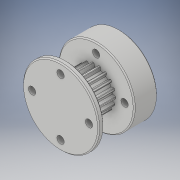
# Autodesk Inventor part: 000.404 - Проставка шкива
Saved by Autodesk Inventor 2019 (Build 230136000, 136)
## iProperties
Created: 2020-03-31
Part Number: 000.404 - Проставка шкива
Material: Типовые
Document SubType Name: Modeling
Designer: Петров Иван
Density: 1 g/cm^3
Appearance: По умолчанию
Author: Петров Иван
Autodesk Inventor part; units mm, degrees
ref_plane "YZ Plane" through (0, 0, 0) normal (1, 0, 0) x (0, 1, 0)
ref_plane "XZ Plane" through (0, 0, 0) normal (0, 1, 0) x (-1, 0, 0)
ref_plane "XY Plane" through (0, 0, 0) normal (0, 0, 1) x (1, 0, 0)
sketch "Эскиз1" plane through (0, 0, 0) normal (0, 0, 1) x (1, 0, 0)
  circle A0 centre (0, -2.75) radius 10.7 projected
  circle A1 centre (0, 5.25) radius 1.025 projected
  circle A2 centre (8, -2.75) radius 1.025 projected
  circle A3 centre (0, -10.75) radius 1.025 projected
  circle A4 centre (-8, -2.75) radius 1.025 projected
  circle A5 centre (0, -2.75) radius 3.05 projected
  point P0 (0, 0)
extrude "Выдавливание1" add sketch "Эскиз1" along normal blind 6.55
sketch "Эскиз2" plane through (0, -2.75, 6.55) normal (0, 0, 1) x (1, 0, 0)
  circle A0 centre (0, 0) radius 7.7
  line L0 (1.9221, 4.23) -> (2.4672, 4.8795)
  arc A1 (2.6243, 4.9099) -> (2.4672, 4.8795) centre (2.5644, 4.7979) ccw
  arc A2 (2.94, 4.7277) -> (2.6243, 4.9099) centre (0, 0) ccw
  arc A3 (2.9922, 4.5764) -> (2.94, 4.7277) centre (2.8729, 4.6198) ccw
  line L1 (2.9922, 4.5764) -> (2.7022, 3.7796)
  line L2 (2.7022, 3.7796) -> (3.2529, 3.3175)
  line L3 (3.2529, 3.3175) -> (3.9873, 3.7415)
  arc A4 (4.1453, 3.7162) -> (3.9873, 3.7415) centre (4.0508, 3.6315) ccw
  arc A5 (4.3796, 3.437) -> (4.1453, 3.7162) centre (0, 0) ccw
  arc A6 (4.377, 3.277) -> (4.3796, 3.437) centre (4.2797, 3.3586) ccw
  line L4 (4.377, 3.277) -> (3.8319, 2.6274)
  line L5 (3.8319, 2.6274) -> (4.1914, 2.0048)
  line L6 (4.1914, 2.0048) -> (5.0265, 2.1521)
  arc A7 (5.1664, 2.0743) -> (5.0265, 2.1521) centre (5.0485, 2.027) ccw
  arc A8 (5.291, 1.7318) -> (5.1664, 2.0743) centre (0, 0) ccw
  arc A9 (5.2338, 1.5823) -> (5.291, 1.7318) centre (5.1703, 1.6923) ccw
  line L7 (5.2338, 1.5823) -> (4.4995, 1.1584)
  line L8 (4.4995, 1.1584) -> (4.6243, 0.4504)
  line L9 (4.6243, 0.4504) -> (5.4594, 0.3032)
  arc A10 (5.5643, 0.1822) -> (5.4594, 0.3032) centre (5.4373, 0.1781) ccw
  arc A11 (5.5643, -0.1822) -> (5.5643, 0.1822) centre (0, 0) ccw
  arc A12 (5.4594, -0.3032) -> (5.5643, -0.1822) centre (5.4373, -0.1781) ccw
  line L10 (5.4594, -0.3032) -> (4.6243, -0.4504)
  line L11 (4.6243, -0.4504) -> (4.4995, -1.1584)
  line L12 (4.4995, -1.1584) -> (5.2338, -1.5823)
  arc A13 (5.291, -1.7318) -> (5.2338, -1.5823) centre (5.1703, -1.6923) ccw
  arc A14 (5.1664, -2.0743) -> (5.291, -1.7318) centre (0, 0) ccw
  arc A15 (5.0265, -2.1521) -> (5.1664, -2.0743) centre (5.0485, -2.027) ccw
  line L13 (5.0265, -2.1521) -> (4.1914, -2.0048)
  line L14 (4.1914, -2.0048) -> (3.8319, -2.6274)
  line L15 (3.8319, -2.6274) -> (4.377, -3.277)
  arc A16 (4.3796, -3.437) -> (4.377, -3.277) centre (4.2797, -3.3586) ccw
  arc A17 (4.1453, -3.7162) -> (4.3796, -3.437) centre (0, 0) ccw
  arc A18 (3.9873, -3.7415) -> (4.1453, -3.7162) centre (4.0508, -3.6315) ccw
  line L16 (3.9873, -3.7415) -> (3.2529, -3.3175)
  line L17 (3.2529, -3.3175) -> (2.7022, -3.7796)
  line L18 (2.7022, -3.7796) -> (2.9922, -4.5764)
  arc A19 (2.94, -4.7277) -> (2.9922, -4.5764) centre (2.8729, -4.6198) ccw
  arc A20 (2.6243, -4.9099) -> (2.94, -4.7277) centre (0, 0) ccw
  arc A21 (2.4672, -4.8795) -> (2.6243, -4.9099) centre (2.5644, -4.7979) ccw
  line L19 (2.4672, -4.8795) -> (1.9221, -4.23)
  line L20 (1.9221, -4.23) -> (1.2466, -4.4758)
  line L21 (1.2466, -4.4758) -> (1.2466, -5.3238)
  arc A22 (1.1457, -5.4481) -> (1.2466, -5.3238) centre (1.1196, -5.3238) ccw
  arc A23 (0.7868, -5.5114) -> (1.1457, -5.4481) centre (0, 0) ccw
  arc A24 (0.6495, -5.4291) -> (0.7868, -5.5114) centre (0.7688, -5.3857) ccw
  line L22 (0.6495, -5.4291) -> (0.3594, -4.6323)
  line L23 (0.3594, -4.6323) -> (-0.3594, -4.6323)
  line L24 (-0.3594, -4.6323) -> (-0.6495, -5.4291)
  arc A25 (-0.7868, -5.5114) -> (-0.6495, -5.4291) centre (-0.7688, -5.3857) ccw
  arc A26 (-1.1457, -5.4481) -> (-0.7868, -5.5114) centre (0, 0) ccw
  arc A27 (-1.2466, -5.3238) -> (-1.1457, -5.4481) centre (-1.1196, -5.3238) ccw
  line L25 (-1.2466, -5.3238) -> (-1.2466, -4.4758)
  line L26 (-1.2466, -4.4758) -> (-1.9221, -4.23)
  line L27 (-1.9221, -4.23) -> (-2.4672, -4.8795)
  arc A28 (-2.6243, -4.9099) -> (-2.4672, -4.8795) centre (-2.5644, -4.7979) ccw
  arc A29 (-2.94, -4.7277) -> (-2.6243, -4.9099) centre (0, 0) ccw
  arc A30 (-2.9922, -4.5764) -> (-2.94, -4.7277) centre (-2.8729, -4.6198) ccw
  line L28 (-2.9922, -4.5764) -> (-2.7022, -3.7796)
  line L29 (-2.7022, -3.7796) -> (-3.2529, -3.3175)
  line L30 (-3.2529, -3.3175) -> (-3.9873, -3.7415)
  arc A31 (-4.1453, -3.7162) -> (-3.9873, -3.7415) centre (-4.0508, -3.6315) ccw
  arc A32 (-4.3796, -3.437) -> (-4.1453, -3.7162) centre (0, 0) ccw
  arc A33 (-4.377, -3.277) -> (-4.3796, -3.437) centre (-4.2797, -3.3586) ccw
  line L31 (-4.377, -3.277) -> (-3.8319, -2.6274)
  line L32 (-3.8319, -2.6274) -> (-4.1914, -2.0048)
  line L33 (-4.1914, -2.0048) -> (-5.0265, -2.1521)
  arc A34 (-5.1664, -2.0743) -> (-5.0265, -2.1521) centre (-5.0485, -2.027) ccw
  arc A35 (-5.291, -1.7318) -> (-5.1664, -2.0743) centre (0, 0) ccw
  arc A36 (-5.2338, -1.5823) -> (-5.291, -1.7318) centre (-5.1703, -1.6923) ccw
  line L34 (-5.2338, -1.5823) -> (-4.4995, -1.1584)
  line L35 (-4.4995, -1.1584) -> (-4.6243, -0.4504)
  line L36 (-4.6243, -0.4504) -> (-5.4594, -0.3032)
  arc A37 (-5.5643, -0.1822) -> (-5.4594, -0.3032) centre (-5.4373, -0.1781) ccw
  arc A38 (-5.5643, 0.1822) -> (-5.5643, -0.1822) centre (0, 0) ccw
  arc A39 (-5.4594, 0.3032) -> (-5.5643, 0.1822) centre (-5.4373, 0.1781) ccw
  line L37 (-5.4594, 0.3032) -> (-4.6243, 0.4504)
  line L38 (-4.6243, 0.4504) -> (-4.4995, 1.1584)
  line L39 (-4.4995, 1.1584) -> (-5.2338, 1.5823)
  arc A40 (-5.291, 1.7318) -> (-5.2338, 1.5823) centre (-5.1703, 1.6923) ccw
  arc A41 (-5.1664, 2.0743) -> (-5.291, 1.7318) centre (0, 0) ccw
  arc A42 (-5.0265, 2.1521) -> (-5.1664, 2.0743) centre (-5.0485, 2.027) ccw
  line L40 (-5.0265, 2.1521) -> (-4.1914, 2.0048)
  line L41 (-4.1914, 2.0048) -> (-3.8319, 2.6274)
  line L42 (-3.8319, 2.6274) -> (-4.377, 3.277)
  arc A43 (-4.3796, 3.437) -> (-4.377, 3.277) centre (-4.2797, 3.3586) ccw
  arc A44 (-4.1453, 3.7162) -> (-4.3796, 3.437) centre (0, 0) ccw
  arc A45 (-3.9873, 3.7415) -> (-4.1453, 3.7162) centre (-4.0508, 3.6315) ccw
  line L43 (-3.9873, 3.7415) -> (-3.2529, 3.3175)
  line L44 (-3.2529, 3.3175) -> (-2.7022, 3.7796)
  line L45 (-2.7022, 3.7796) -> (-2.9922, 4.5764)
  arc A46 (-2.94, 4.7277) -> (-2.9922, 4.5764) centre (-2.8729, 4.6198) ccw
  arc A47 (-2.6243, 4.9099) -> (-2.94, 4.7277) centre (0, 0) ccw
  arc A48 (-2.4672, 4.8795) -> (-2.6243, 4.9099) centre (-2.5644, 4.7979) ccw
  line L46 (-2.4672, 4.8795) -> (-1.9221, 4.23)
  line L47 (-1.9221, 4.23) -> (-1.2466, 4.4758)
  line L48 (-1.2466, 4.4758) -> (-1.2466, 5.3238)
  arc A49 (-1.1457, 5.4481) -> (-1.2466, 5.3238) centre (-1.1196, 5.3238) ccw
  arc A50 (-0.7868, 5.5114) -> (-1.1457, 5.4481) centre (0, 0) ccw
  arc A51 (-0.6495, 5.4291) -> (-0.7868, 5.5114) centre (-0.7688, 5.3857) ccw
  line L49 (-0.6495, 5.4291) -> (-0.3594, 4.6323)
  line L50 (-0.3594, 4.6323) -> (0.3594, 4.6323)
  line L51 (0.3594, 4.6323) -> (0.6495, 5.4291)
  arc A52 (0.7868, 5.5114) -> (0.6495, 5.4291) centre (0.7688, 5.3857) ccw
  arc A53 (1.1457, 5.4481) -> (0.7868, 5.5114) centre (0, 0) ccw
  arc A54 (1.2466, 5.3238) -> (1.1457, 5.4481) centre (1.1196, 5.3238) ccw
  line L52 (1.2466, 5.3238) -> (1.2466, 4.4758)
  line L53 (1.2466, 4.4758) -> (1.9221, 4.23)
  circle A55 centre (0, 0) radius 7.7
  circle A56 centre (0, 0) radius 8
  point P0 (0, 2.75)
  constraints: 108 end point, 108 point on circle, 57 centre point
extrude "Выдавливание2" add sketch "Эскиз2" along normal blind 8.5 contours L0 A1 A2 A3 L1 L2 L3 A4 A5 A6 L4 L5 L6 A7 A8 A9 L7 L8 L9 A10 A11 A12 L10 L11 L12 A13 A14 A15 L13 L14 L15 A16 A17 A18 L16 L17 L18 A19 A20 A21 L19 L20 L21 A22 A23 A24 L22 L23 L24 A25 A26 A27 L25 L26 L27 A28 A29 A30 L28 L29 L30 A31 A32 A33 L31 L32 L33 A34 A35 A36 L34 L35 L36 A37 A38 A39 L37 L38 L39 A40 A41 A42 L40 L41 L42 A43 A44 A45 L43 L44 L45 A46 A47 A48 L46 L47 L48 A49 A50 A51 L49 L50 L51 A52 A53 A54 L52 L53
sketch "Эскиз3" plane through (0, -2.75, 15.05) normal (0, 0, 1) x (1, 0, 0)
  circle A0 centre (0, 0) radius 10.7 projected
  circle A1 centre (0, 0) radius 10.7
  point P0 (0, 2.75)
  constraints: 1 centre point, 1 coincident
extrude "Выдавливание3" add sketch "Эскиз3" along normal blind 1.5
chamfer "Фаска1" distance 0.3 angle 45 4 edges at (-10.7, -2.75, 15.05) (-10.7, -2.75, 16.55) (-10.7, -2.75, 6.55) (-10.7, -2.75, 0)
sketch "Эскиз4" plane through (0, -2.75, 16.55) normal (0, 0, 1) x (1, 0, 0)
  circle A0 centre (0, 8) radius 1.025 projected
  circle A1 centre (-8, 0) radius 1.025 projected
  circle A2 centre (8, 0) radius 1.025 projected
  circle A3 centre (0, -8) radius 1.025 projected
  point P0 (0, 2.75)
extrude "Выдавливание4" cut sketch "Эскиз4" against normal blind 2
